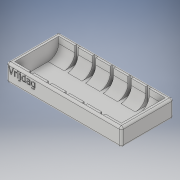
# Autodesk Inventor part: bakje woensdag
Saved by Autodesk Inventor 2019 (Build 230136000, 136)
## iProperties
Created: 2020-10-20
Part Number: bakje woensdag
Material: Generic
Document SubType Name: Modeling
Designer: daanswinters
Density: 1 g/cm^3
Appearance: Default
Author: daanswinters
Autodesk Inventor part; units mm, degrees
ref_plane "YZ Plane" through (0, 0, 0) normal (1, 0, 0) x (0, 1, 0)
ref_plane "XZ Plane" through (0, 0, 0) normal (0, 1, 0) x (-1, 0, 0)
ref_plane "XY Plane" through (0, 0, 0) normal (0, 0, 1) x (1, 0, 0)
sketch "Sketch1" plane through (0, 0, 0) normal (0, 0, 1) x (1, 0, 0)
  line L0 (55, -8.5) -> (-55, -8.5)
  line L1 (-55, -8.5) -> (-55, 8.5)
  line L2 (-55, 8.5) -> (55, 8.5)
  line L3 (55, 8.5) -> (55, -8.5)
  line L4 (55, -8.5) -> (-55, 8.5) construction
  line L5 (-55, -8.5) -> (55, 8.5) construction
  point P0 (0, 0)
  dimension "d0" = 110
  dimension "d1" = 17
  constraints: 12 end point, 2 midpoint, 2 parallel, 1 horizontal, 1 perpendicular
  measures "d0" distance of L1.end L2.end
  measures "d1" distance of L0.end L1.end
extrude "Extrusion1" add sketch "Sketch1" along normal blind 50
sketch "Sketch2" plane through (-55, 8.5, 0) normal (0, 1, 0) x (1, 0, 0)
  line L0 (0, 0) -> (0, -50) projected
  line L1 (110, -50) -> (0, -50)
  line L2 (0, -50) -> (0, 0)
  line L3 (0, 0) -> (110, 0)
  line L4 (110, 0) -> (110, -50)
  line L5 (110, -50) -> (0, 0) construction
  line L6 (0, -50) -> (110, 0) construction
  line L7 (106, -46) -> (106, -4)
  line L8 (4, -4) -> (4, -46)
  line L9 (56.15, -2) -> (53.85, -2)
  line L10 (53.85, -48) -> (56.15, -48)
  line L11 (56.15, -2) -> (53.85, -48) construction
  line L12 (53.85, -2) -> (56.15, -48) construction
  line L13 (73.15, -2) -> (70.85, -2)
  line L14 (70.85, -48) -> (73.15, -48)
  line L15 (73.15, -2) -> (70.85, -48) construction
  line L16 (70.85, -2) -> (73.15, -48) construction
  line L17 (0, -25) -> (110, -25) construction
  line L18 (87.85, -2) -> (90.15, -2)
  line L19 (90.15, -48) -> (87.85, -48)
  line L20 (87.85, -2) -> (90.15, -48) construction
  line L21 (90.15, -2) -> (87.85, -48) construction
  line L22 (36.85, -2) -> (39.15, -2)
  line L23 (39.15, -48) -> (36.85, -48)
  line L24 (36.85, -2) -> (39.15, -48) construction
  line L25 (39.15, -2) -> (36.85, -48) construction
  line L26 (19.85, -2) -> (22.15, -2)
  line L27 (22.15, -48) -> (19.85, -48)
  line L28 (19.85, -2) -> (22.15, -48) construction
  line L29 (22.15, -2) -> (19.85, -48) construction
  line L30 (90.15, -2) -> (90.15, -4)
  line L31 (90.15, -46) -> (90.15, -48)
  line L32 (87.85, -48) -> (87.85, -46)
  line L33 (87.85, -4) -> (87.85, -2)
  line L34 (73.15, -48) -> (73.15, -46)
  line L35 (73.15, -4) -> (73.15, -2)
  line L36 (70.85, -2) -> (70.85, -4)
  line L37 (70.85, -46) -> (70.85, -48)
  line L38 (56.15, -4) -> (56.15, -2)
  line L39 (53.85, -2) -> (53.85, -4)
  line L40 (53.85, -46) -> (53.85, -48)
  line L41 (56.15, -48) -> (56.15, -46)
  line L42 (39.15, -2) -> (39.15, -4)
  line L43 (39.15, -46) -> (39.15, -48)
  line L44 (36.85, -48) -> (36.85, -46)
  line L45 (36.85, -4) -> (36.85, -2)
  line L46 (22.15, -2) -> (22.15, -4)
  line L47 (19.85, -48) -> (19.85, -46)
  line L48 (19.85, -4) -> (19.85, -2)
  line L49 (22.15, -46) -> (22.15, -48)
  line L50 (4, -46) -> (19.95, -46)
  line L51 (22.05, -46) -> (36.95, -46)
  line L52 (39.05, -46) -> (53.95, -46)
  line L53 (56.05, -46) -> (70.95, -46)
  line L54 (73.05, -46) -> (87.95, -46)
  line L55 (90.05, -46) -> (106, -46)
  line L56 (106, -4) -> (90.05, -4)
  line L57 (87.95, -4) -> (73.05, -4)
  line L58 (70.95, -4) -> (56.05, -4)
  line L59 (53.95, -4) -> (39.05, -4)
  line L60 (36.95, -4) -> (22.05, -4)
  line L61 (19.95, -4) -> (4, -4)
  point P0 (55, 0)
  point P1 (55, -25)
  point P2 (72, -25)
  point P3 (89, -25)
  point P4 (38, -25)
  point P5 (21, -25)
  dimension "d4" = 65.556
  dimension "d5" = 110
  dimension "d7" = 2.3
  dimension "d8" = 46
  dimension "d9" = 2.3
  dimension "d10" = 46
  dimension "d11" = 0
  dimension "d12" = 2.3
  dimension "d13" = 46
  dimension "d14" = 2.3
  dimension "d15" = 46
  dimension "d16" = 2.3
  dimension "d17" = 46
  dimension "d18" = 17
  dimension "d19" = 17
  dimension "d20" = 17
  dimension "d21" = 17
  dimension "d22" = 2.862
  dimension "d23" = 2.862
  dimension "d24" = 106
  dimension "d25" = 4
  dimension "d26" = 42
  dimension "d27" = 2
  dimension "d28" = 0
  dimension "d29" = 42
  dimension "d30" = 0
  dimension "d31" = 42
  dimension "d32" = 0
  dimension "d33" = 42
  dimension "d34" = 0
  dimension "d35" = 42
  dimension "d36" = 0
  dimension "d37" = 42
  constraints: 122 end point, 73 parallel, 43 point on line, 17 perpendicular, 14 midpoint, 6 horizontal
  measures "d4" angle of L5 L0
  measures "d5" distance between parallel lines of L4 L0
  measures "d7" distance of L10.end L10.start
  measures "d8" distance of L10.start L9.end
  measures "d9" distance of L14.end L14.start
  measures "d10" distance of L14.start L13.end
  measures "d11" distance from line of L17 point (72, -25)
  measures "d12" distance of L19.start L19.end
  measures "d13" distance of L18.end L19.start
  measures "d14" distance of L23.start L23.end
  measures "d15" distance of L22.end L23.start
  measures "d16" distance of L27.start L27.end
  measures "d17" distance of L26.end L27.start
  measures "d18" distance of point (72, -25) point (55, -25)
  measures "d19" distance of point (89, -25) point (72, -25)
  measures "d20" distance of point (38, -25) point (55, -25)
  measures "d21" distance of point (21, -25) point (38, -25)
  measures "d22" angle of L0 L20
  measures "d23" angle of L0 L21
  measures "d24" distance between parallel lines of L7 L0
  measures "d25" distance between parallel lines of L8 L0
  measures "d26" distance between parallel lines of L56 L55
  measures "d27" distance between parallel lines of L56 L18
  measures "d28" distance between parallel lines of L56 L57
  measures "d29" distance between parallel lines of L56 L54
  measures "d30" distance between parallel lines of L56 L58
  measures "d31" distance between parallel lines of L56 L53
  measures "d32" distance between parallel lines of L56 L59
  measures "d33" distance between parallel lines of L56 L52
  measures "d34" distance between parallel lines of L56 L60
  measures "d35" distance between parallel lines of L56 L51
  measures "d36" distance between parallel lines of L56 L61
  measures "d37" distance between parallel lines of L56 L50
extrude "Extrusion2" cut sketch "Sketch2" against normal blind 16 contours L55 L31 L19 L32 L54 L34 L14 L37 L53 L41 L10 L40 L52 L43 L23 L44 L51 L49 L27 L47 L50 L8 L61 L48 L26 L46 L60 L45 L22 L42 L59 L39 L9 L38 L58 L36 L13 L35 L57 L33 L18 L30 L56 L7
fillet "Fillet1" radius 2 12 edges at (-55, 0, 50) (-55, 0, 0) (55, 0, 50) (55, 0, 0) (0, 8.5, 50) (-55, 8.5, 25) (0, 8.5, 0) (55, 8.5, 25) (55, -8.5, 25) (0, -8.5, 50) (-55, -8.5, 25) (0, -8.5, 0)
fillet "Fillet2" radius 10 6 edges at (-43.075, -7.5, 4) (-25.5, -7.5, 4) (-8.5, -7.5, 4) (8.5, -7.5, 4) (25.5, -7.5, 4) (43.075, -7.5, 4)
sketch "Sketch3" plane through (35.15, 8.5, 4) normal (0, 1, 0) x (1, 0, 0)
  line L0 (-70.3, -44) -> (-70.3, -42) projected
  line L1 (-51, 2) -> (-53.3, 2)
  line L2 (-34, 2) -> (-34, 0) projected
  line L3 (-36.3, -44) -> (-36.3, -42) projected
  line L4 (-19.3, -44) -> (-19.3, -42) projected
  line L5 (-2.3, -44) -> (-2.3, -42) projected
  line L6 (0, 2) -> (0, 0) projected
  line L7 (-19.8, 2) -> (-16.5, 2)
  line L8 (-16.5, 2) -> (-16.5, -44)
  line L9 (-16.5, -44) -> (-19.8, -44)
  line L10 (-19.8, -44) -> (-19.8, 2)
  line L11 (-19.8, 2) -> (-16.5, -44) construction
  line L12 (-16.5, 2) -> (-19.8, -44) construction
  line L13 (-2.8, -44) -> (0.5, -44)
  line L14 (0.5, -44) -> (0.5, 2)
  line L15 (0.5, 2) -> (-2.8, 2)
  line L16 (-2.8, 2) -> (-2.8, -44)
  line L17 (-2.8, -44) -> (0.5, 2) construction
  line L18 (0.5, -44) -> (-2.8, 2) construction
  line L19 (-36.8, -44) -> (-33.5, -44)
  line L20 (-33.5, -44) -> (-33.5, 2)
  line L21 (-33.5, 2) -> (-36.8, 2)
  line L22 (-36.8, 2) -> (-36.8, -44)
  line L23 (-36.8, -44) -> (-33.5, 2) construction
  line L24 (-33.5, -44) -> (-36.8, 2) construction
  line L25 (-51, 2) -> (-36.3, 2) projected
  line L26 (-53.8, -44) -> (-50.5, -44)
  line L27 (-50.5, -44) -> (-50.5, 2)
  line L28 (-50.5, 2) -> (-53.8, 2)
  line L29 (-53.8, 2) -> (-53.8, -44)
  line L30 (-53.8, -44) -> (-50.5, 2) construction
  line L31 (-50.5, -44) -> (-53.8, 2) construction
  line L32 (-53.3, -44) -> (-68, -44) projected
  line L33 (-70.8, 2) -> (-67.5, 2)
  line L34 (-67.5, 2) -> (-67.5, -44)
  line L35 (-67.5, -44) -> (-70.8, -44)
  line L36 (-70.8, -44) -> (-70.8, 2)
  line L37 (-70.8, 2) -> (-67.5, -44) construction
  line L38 (-67.5, 2) -> (-70.8, -44) construction
  point P0 (-35.15, 4)
  point P1 (-68, 2)
  point P2 (-17, 2)
  point P3 (-18.15, -21)
  point P4 (-1.15, -21)
  point P5 (-35.15, -21)
  point P6 (-52.15, -21)
  point P7 (-69.15, -21)
  dimension "d42" = 3.3
  dimension "d43" = 46
  dimension "d44" = 3.3
  dimension "d45" = 3.3
  dimension "d46" = 3.3
  dimension "d47" = 3.3
  dimension "d48" = 90
  dimension "d49" = 0.5
  dimension "d50" = 16.5
  dimension "d51" = 33.5
  dimension "d52" = 50.5
  dimension "d53" = 67.5
  dimension "d54" = 46
  dimension "d55" = 0
  dimension "d56" = 53.3
  constraints: 62 end point, 14 parallel, 10 midpoint, 5 horizontal, 5 perpendicular, 3 point on line
  measures "d42" distance of L8.end L9.end
  measures "d43" distance of L7.end L8.end
  measures "d44" distance of L15.end L14.end
  measures "d45" distance of L21.end L20.end
  measures "d46" distance of L28.end L27.end
  measures "d47" distance of L34.end L35.end
  measures "d48" angle of L6 L1
  measures "d49" distance between parallel lines of L6 L14
  measures "d50" distance between parallel lines of L6 L8
  measures "d51" distance between parallel lines of L6 L20
  measures "d52" distance between parallel lines of L6 L27
  measures "d53" distance between parallel lines of L6 L34
  measures "d54" distance between parallel lines of L25 L9
  measures "d55" distance between parallel lines of L15 L25
  measures "d56" distance from line of L1.end L6
extrude "Extrusion3" cut sketch "Sketch3" against normal blind 16
sketch "Sketch4" plane through (0, 0, 50) normal (0, 0, 1) x (1, 0, 0)
  line L0 (-52.9749, 6.5012) -> (53.0345, 6.5012) construction
  line L1 (53.0345, 6.5012) -> (53.0345, -6.5247) construction
  line L2 (53.0345, -6.5247) -> (-52.9749, -6.5247) construction
  line L3 (-52.9749, -6.5247) -> (-52.9749, 6.5012) construction
  line L4 (-47.9328, 6.2294) -> (-50.0337, 0.1294)
  line L5 (-50.0337, 0.1294) -> (-50.9086, 0.1294)
  line L6 (-50.9086, 0.1294) -> (-53.0095, 6.2294)
  line L7 (-53.0095, 6.2294) -> (-52.1395, 6.2294)
  line L8 (-52.1395, 6.2294) -> (-50.4489, 1.1625)
  line L9 (-50.4489, 1.1625) -> (-48.7583, 6.2294)
  line L10 (-48.7583, 6.2294) -> (-47.9328, 6.2294)
  line L11 (-44.9817, 3.8813) -> (-45.0212, 3.8813)
  spline S0 degree 2 poles (-45.0212, 3.8813) (-45.1102, 3.906) (-45.303, 3.9159) (-45.4364, 3.9159) knots 0 0 0 1 2 2 2
  spline S1 degree 2 poles (-45.4364, 3.9159) (-45.7479, 3.9159) (-46.3608, 3.644) (-46.6376, 3.3771) knots 0 0 0 1 2 2 2
  line L12 (-46.6376, 3.3771) -> (-46.6376, 0.1294)
  line L13 (-46.6376, 0.1294) -> (-47.4088, 0.1294)
  line L14 (-47.4088, 0.1294) -> (-47.4088, 4.7068)
  line L15 (-47.4088, 4.7068) -> (-46.6376, 4.7068)
  line L16 (-46.6376, 4.7068) -> (-46.6376, 4.0247)
  spline S2 degree 2 poles (-46.6376, 4.0247) (-46.2175, 4.4004) (-45.5897, 4.7068) (-45.2931, 4.7068) knots 0 0 0 1 2 2 2
  spline S3 degree 2 poles (-45.2931, 4.7068) (-45.1744, 4.7068) (-45.0558, 4.697) (-44.9817, 4.6821) knots 0 0 0 1 2 2 2
  line L17 (-44.9817, 4.6821) -> (-44.9817, 3.8813)
  line L18 (-43.5975, 0.1294) -> (-44.3687, 0.1294)
  line L19 (-44.3687, 0.1294) -> (-44.3687, 4.7068)
  line L20 (-44.3687, 4.7068) -> (-43.5975, 4.7068)
  line L21 (-43.5975, 4.7068) -> (-43.5975, 0.1294)
  line L22 (-43.5432, 5.4681) -> (-44.4181, 5.4681)
  line L23 (-44.4181, 5.4681) -> (-44.4181, 6.2689)
  line L24 (-44.4181, 6.2689) -> (-43.5432, 6.2689)
  line L25 (-43.5432, 6.2689) -> (-43.5432, 5.4681)
  spline S4 degree 2 poles (-41.2198, 0.0008) (-41.2198, -0.7802) (-42.0602, -1.6008) (-42.7967, -1.6008) knots 0 0 0 1 2 2 2
  spline S5 degree 2 poles (-42.7967, -1.6008) (-42.9253, -1.6008) (-43.2416, -1.5761) (-43.3949, -1.5513) knots 0 0 0 1 2 2 2
  line L26 (-43.3949, -1.5513) -> (-43.3949, -0.8593)
  line L27 (-43.3949, -0.8593) -> (-43.3504, -0.8593)
  spline S6 degree 2 poles (-43.3504, -0.8593) (-43.2614, -0.8791) (-43.0439, -0.9186) (-42.945, -0.9186) knots 0 0 0 1 2 2 2
  spline S7 degree 2 poles (-42.945, -0.9186) (-42.6385, -0.9186) (-42.2381, -0.7654) (-42.1442, -0.6022) knots 0 0 0 1 2 2 2
  spline S8 degree 2 poles (-42.1442, -0.6022) (-42.0503, -0.4539) (-41.991, -0.0041) (-41.991, 0.3172) knots 0 0 0 1 2 2 2
  line L28 (-41.991, 0.3172) -> (-41.991, 4.0692)
  line L29 (-41.991, 4.0692) -> (-42.8165, 4.0692)
  line L30 (-42.8165, 4.0692) -> (-42.8165, 4.7068)
  line L31 (-42.8165, 4.7068) -> (-41.2198, 4.7068)
  line L32 (-41.2198, 4.7068) -> (-41.2198, 0.0008)
  line L33 (-41.2149, 5.4681) -> (-42.0898, 5.4681)
  line L34 (-42.0898, 5.4681) -> (-42.0898, 6.2689)
  line L35 (-42.0898, 6.2689) -> (-41.2149, 6.2689)
  line L36 (-41.2149, 6.2689) -> (-41.2149, 5.4681)
  line L37 (-36.583, 0.1294) -> (-37.3542, 0.1294)
  line L38 (-37.3542, 0.1294) -> (-37.3542, 0.594)
  spline S9 degree 2 poles (-37.3542, 0.594) (-37.5321, 0.4457) (-37.7941, 0.248) (-37.9721, 0.164) knots 0 0 0 1 2 2 2
  spline S10 degree 2 poles (-37.9721, 0.164) (-38.1352, 0.0849) (-38.4862, 0.0008) (-38.7185, 0.0008) knots 0 0 0 1 2 2 2
  spline S11 degree 2 poles (-38.7185, 0.0008) (-39.0942, 0.0008) (-39.727, 0.3123) (-39.9494, 0.6138) knots 0 0 0 1 2 2 2
  spline S12 degree 2 poles (-39.9494, 0.6138) (-40.1718, 0.9153) (-40.419, 1.8051) (-40.419, 2.3835) knots 0 0 0 1 2 2 2
  spline S13 degree 2 poles (-40.419, 2.3835) (-40.419, 2.9866) (-40.1076, 3.8665) (-39.8357, 4.1977) knots 0 0 0 1 2 2 2
  spline S14 degree 2 poles (-39.8357, 4.1977) (-39.5836, 4.4943) (-38.8767, 4.8354) (-38.4862, 4.8354) knots 0 0 0 1 2 2 2
  spline S15 degree 2 poles (-38.4862, 4.8354) (-38.1451, 4.8354) (-37.6359, 4.6821) (-37.3542, 4.5239) knots 0 0 0 1 2 2 2
  line L39 (-37.3542, 4.5239) -> (-37.3542, 6.5012)
  line L40 (-37.3542, 6.5012) -> (-36.583, 6.5012)
  line L41 (-36.583, 6.5012) -> (-36.583, 0.1294)
  line L42 (-37.3542, 1.2416) -> (-37.3542, 3.8863)
  spline S16 degree 2 poles (-37.3542, 3.8863) (-37.6409, 4.0247) (-38.0957, 4.1285) (-38.3577, 4.1285) knots 0 0 0 1 2 2 2
  spline S17 degree 2 poles (-38.3577, 4.1285) (-38.9509, 4.1285) (-39.6231, 3.2387) (-39.6231, 2.3983) knots 0 0 0 1 2 2 2
  spline S18 degree 2 poles (-39.6231, 2.3983) (-39.6231, 1.5876) (-39.109, 0.7324) (-38.5406, 0.7324) knots 0 0 0 1 2 2 2
  spline S19 degree 2 poles (-38.5406, 0.7324) (-38.239, 0.7324) (-37.6261, 1.0093) (-37.3542, 1.2416) knots 0 0 0 1 2 2 2
  spline S20 degree 2 poles (-32.9151, 0.6138) (-33.009, 0.5446) (-33.3254, 0.2974) (-33.4737, 0.2233) knots 0 0 0 1 2 2 2
  spline S21 degree 2 poles (-33.4737, 0.2233) (-33.6764, 0.1145) (-34.057, 0.0008) (-34.403, 0.0008) knots 0 0 0 1 2 2 2
  spline S22 degree 2 poles (-34.403, 0.0008) (-34.6848, 0.0008) (-35.194, 0.2134) (-35.3868, 0.4062) knots 0 0 0 1 2 2 2
  spline S23 degree 2 poles (-35.3868, 0.4062) (-35.5697, 0.594) (-35.7921, 1.1477) (-35.7921, 1.4542) knots 0 0 0 1 2 2 2
  spline S24 degree 2 poles (-35.7921, 1.4542) (-35.7921, 1.9287) (-35.3917, 2.601) (-34.9567, 2.7938) knots 0 0 0 1 2 2 2
  spline S25 degree 2 poles (-34.9567, 2.7938) (-34.5711, 2.9718) (-33.5231, 3.1052) (-32.9151, 3.1398) knots 0 0 0 1 2 2 2
  line L43 (-32.9151, 3.1398) -> (-32.9151, 3.2881)
  spline S26 degree 2 poles (-32.9151, 3.2881) (-32.9151, 3.5551) (-33.0782, 3.8863) (-33.2265, 3.9802) knots 0 0 0 1 2 2 2
  spline S27 degree 2 poles (-33.2265, 3.9802) (-33.3748, 4.0741) (-33.8, 4.1334) (-34.0274, 4.1334) knots 0 0 0 1 2 2 2
  spline S28 degree 2 poles (-34.0274, 4.1334) (-34.2943, 4.1334) (-35.016, 3.9752) (-35.3769, 3.822) knots 0 0 0 1 2 2 2
  line L44 (-35.3769, 3.822) -> (-35.4214, 3.822)
  line L45 (-35.4214, 3.822) -> (-35.4214, 4.608)
  spline S29 degree 2 poles (-35.4214, 4.608) (-35.2088, 4.6673) (-34.4129, 4.8156) (-34.0224, 4.8156) knots 0 0 0 1 2 2 2
  spline S30 degree 2 poles (-34.0224, 4.8156) (-33.5479, 4.8156) (-32.9003, 4.6673) (-32.6432, 4.4745) knots 0 0 0 1 2 2 2
  spline S31 degree 2 poles (-32.6432, 4.4745) (-32.3911, 4.2867) (-32.144, 3.6885) (-32.144, 3.2585) knots 0 0 0 1 2 2 2
  line L46 (-32.144, 3.2585) -> (-32.144, 0.1294)
  line L47 (-32.144, 0.1294) -> (-32.9151, 0.1294)
  line L48 (-32.9151, 0.1294) -> (-32.9151, 0.6138)
  line L49 (-32.9151, 1.2564) -> (-32.9151, 2.5269)
  spline S32 degree 2 poles (-32.9151, 2.5269) (-33.1919, 2.5021) (-34.0274, 2.4181) (-34.2894, 2.339) knots 0 0 0 1 2 2 2
  spline S33 degree 2 poles (-34.2894, 2.339) (-34.5958, 2.2451) (-34.9962, 1.8546) (-34.9962, 1.5085) knots 0 0 0 1 2 2 2
  spline S34 degree 2 poles (-34.9962, 1.5085) (-34.9962, 1.1131) (-34.5513, 0.7127) (-34.1262, 0.7127) knots 0 0 0 1 2 2 2
  spline S35 degree 2 poles (-34.1262, 0.7127) (-33.7654, 0.7127) (-33.1722, 1.0241) (-32.9151, 1.2564) knots 0 0 0 1 2 2 2
  spline S36 degree 2 poles (-30.8983, -0.6022) (-30.8192, -0.6368) (-30.5176, -0.7456) (-30.3248, -0.7901) knots 0 0 0 1 2 2 2
  spline S37 degree 2 poles (-30.3248, -0.7901) (-30.1123, -0.8445) (-29.7514, -0.9087) (-29.5389, -0.9087) knots 0 0 0 1 2 2 2
  spline S38 degree 2 poles (-29.5389, -0.9087) (-29.1829, -0.9087) (-28.6886, -0.7209) (-28.5502, -0.5528) knots 0 0 0 1 2 2 2
  spline S39 degree 2 poles (-28.5502, -0.5528) (-28.4167, -0.3847) (-28.3129, 0.0552) (-28.3129, 0.337) knots 0 0 0 1 2 2 2
  line L50 (-28.3129, 0.337) -> (-28.3129, 0.7374)
  spline S40 degree 2 poles (-28.3129, 0.7374) (-28.6244, 0.4655) (-29.2225, 0.2085) (-29.6723, 0.2085) knots 0 0 0 1 2 2 2
  spline S41 degree 2 poles (-29.6723, 0.2085) (-30.4534, 0.2085) (-31.3778, 1.3701) (-31.3778, 2.4626) knots 0 0 0 1 2 2 2
  spline S42 degree 2 poles (-31.3778, 2.4626) (-31.3778, 3.0311) (-31.0564, 3.911) (-30.7895, 4.2224) knots 0 0 0 1 2 2 2
  spline S43 degree 2 poles (-30.7895, 4.2224) (-30.5325, 4.5141) (-29.8256, 4.8354) (-29.4499, 4.8354) knots 0 0 0 1 2 2 2
  spline S44 degree 2 poles (-29.4499, 4.8354) (-29.094, 4.8354) (-28.5749, 4.6673) (-28.3129, 4.5141) knots 0 0 0 1 2 2 2
  line L51 (-28.3129, 4.5141) -> (-28.2684, 4.7068)
  line L52 (-28.2684, 4.7068) -> (-27.5418, 4.7068)
  line L53 (-27.5418, 4.7068) -> (-27.5418, 0.6534)
  spline S45 degree 2 poles (-27.5418, 0.6534) (-27.5418, -0.5133) (-28.5552, -1.6008) (-29.5982, -1.6008) knots 0 0 0 1 2 2 2
  spline S46 degree 2 poles (-29.5982, -1.6008) (-29.9343, -1.6008) (-30.6363, -1.492) (-30.9378, -1.403) knots 0 0 0 1 2 2 2
  line L54 (-30.9378, -1.403) -> (-30.9378, -0.6022)
  line L55 (-30.9378, -0.6022) -> (-30.8983, -0.6022)
  line L56 (-28.3129, 1.3701) -> (-28.3129, 3.8863)
  spline S47 degree 2 poles (-28.3129, 3.8863) (-28.5996, 4.0247) (-29.0841, 4.1433) (-29.3263, 4.1433) knots 0 0 0 1 2 2 2
  spline S48 degree 2 poles (-29.3263, 4.1433) (-29.9096, 4.1433) (-30.5819, 3.2832) (-30.5819, 2.4774) knots 0 0 0 1 2 2 2
  spline S49 degree 2 poles (-30.5819, 2.4774) (-30.5819, 1.7162) (-30.0727, 0.9203) (-29.4993, 0.9203) knots 0 0 0 1 2 2 2
  spline S50 degree 2 poles (-29.4993, 0.9203) (-29.1978, 0.9203) (-28.565, 1.1576) (-28.3129, 1.3701) knots 0 0 0 1 2 2 2
  point P0 (0, 0)
  constraints: 2 other
extrude "Extrusion4" cut sketch "Sketch4" against normal blind 0.5
fillet "Fillet3" radius 10 6 edges at (-43.325, -7.5, 46) (-25.5, -7.5, 46) (-8.5, -7.5, 46) (8.5, -7.5, 46) (25.5, -7.5, 46) (43.325, -7.5, 46)
body "Solid1"
